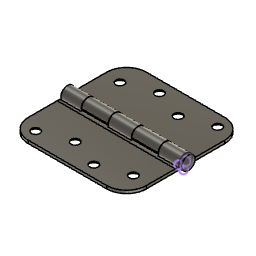
Example - Hinge v2 (Autodesk Fusion 360 design; units mm, degrees)
Autodesk Fusion 360 part; units mm, degrees
sketch "Sketch1" plane through (0, 0, 0) normal (1, 0, 0) x (0, 1, 0)
  line L0 (-56.0607, 28.9615) -> (-14.2484, 28.9615)
  line L1 (-9.4019, 28.157) -> (-6.4108, 27.1358)
  arc A0 (-6.4108, 27.1358) -> (-8.6089, 30.3207) centre (-5.3607, 30.2115) ccw
  circle A1 centre (-5.3607, 30.2115) radius 2.75
  line L2 (-56.0607, 26.4615) -> (-14.2484, 26.4615)
  line L3 (-10.2097, 25.791) -> (-7.2185, 24.7698)
  arc A2 (-7.2185, 24.7698) -> (-11.1075, 30.4047) centre (-5.3607, 30.2115) ccw
  line L4 (-56.0607, 28.9615) -> (-56.0607, 26.4615)
  line L5 (-11.1075, 30.4047) -> (-11.1411, 29.4053)
  line L6 (-11.1411, 29.4053) -> (-8.6425, 29.3212)
  line L7 (-8.6425, 29.3212) -> (-8.6089, 30.3207)
  arc A3 (-9.4019, 28.157) -> (-14.2484, 28.9615) centre (-14.2484, 13.9615) ccw
  arc A4 (-10.2097, 25.791) -> (-14.2484, 26.4615) centre (-14.2484, 13.9615) ccw
  line L8 (14.6393, 52.3652) -> (14.6393, 9.6795) construction
  arc A5 (40.386, 30.4047) -> (36.497, 24.7698) centre (34.6393, 30.2115) ccw
  circle A6 centre (34.6393, 30.2115) radius 2.75
  line L9 (85.3393, 28.9615) -> (43.5269, 28.9615)
  line L10 (85.3393, 28.9615) -> (85.3393, 26.4615)
  arc A7 (43.5269, 28.9615) -> (38.6804, 28.157) centre (43.5269, 13.9615) ccw
  line L11 (40.386, 30.4047) -> (40.4196, 29.4053)
  arc A8 (37.8874, 30.3207) -> (35.6893, 27.1358) centre (34.6393, 30.2115) ccw
  line L12 (38.6804, 28.157) -> (35.6893, 27.1358)
  line L13 (40.4196, 29.4053) -> (37.921, 29.3212)
  line L14 (39.4882, 25.791) -> (36.497, 24.7698)
  line L15 (85.3393, 26.4615) -> (43.5269, 26.4615)
  arc A9 (43.5269, 26.4615) -> (39.4882, 25.791) centre (43.5269, 13.9615) ccw
  line L16 (37.921, 29.3212) -> (37.8874, 30.3207)
  dimension "d1" = 5.5
  dimension "d3" = 50.7
  dimension "d4" = 2.5
  dimension "d5" = 1.25
  dimension "d6" = 0.5
  dimension "d7" = 2.5
  dimension "d9" = 1
  dimension "d10" = 15
  dimension "d12" = 20
  constraint tangent L1 A0
  constraint parallel L0 L2
  constraint parallel L1 L3
  constraint concentric A0 A2
  constraint tangent L3 A2
  constraint concentric A0 A1
  constraint horizontal L0
  constraint perpendicular L2 L4
  constraint tangent A2 L5
  constraint perpendicular L5 L6
  constraint perpendicular L6 L7
  constraint tangent A0 L7
  constraint tangent L0 A3
  constraint tangent L1 A3
  constraint tangent L2 A4
  constraint tangent L3 A4
  constraint concentric A3 A4
  constraint vertical L8
  constraint symmetric L0.start L8 L9.start
  constraint symmetric L1.end L8 A8.end
  constraint symmetric A0.end L8 A8.start
  constraint symmetric A0 L8 A8
  constraint symmetric A1 L8 A6
  constraint symmetric L2.start L8 L10.end
  constraint symmetric L3.end L8 A5.end
  constraint symmetric A2.end L8 A5.start
  constraint symmetric A2 L8 A5
  constraint symmetric L5.end L8 L11.end
  constraint symmetric L6.end L8 L13.end
  constraint symmetric L0.end L8 L9.end
  constraint symmetric L1.start L8 A7.end
  constraint symmetric A3 L8 A7
  constraint symmetric L2.end L8 L15.end
  constraint symmetric L3.start L8 L14.start
  constraint symmetric A4 L8 A9
  measures "d1" diameter of A1
  measures "d3" distance of A0.centre L4
  measures "d4" distance of L0 L2
  measures "d5" distance of L0 A0.centre
  measures "d6" distance of A0 A1
  measures "d7" distance of L1 L3
  measures "d9" distance of A2.end L6
  measures "d10" radius of A3
  measures "d12" distance of A0.centre L8
extrude "Extrude1" add sketch "Sketch1" along normal blind 101.4 contours L0 L1 A0 L2 L3 A2 L4 L5 L6 L7 A3 A4 makes body 1 in component "Hinge side 1"
sketch "Sketch1 (2)" plane through (0, 0, 28.9615) normal (0, 0, 1) x (-1, 0, 0) in component "Hinge side 1"
  line L0 (0, 14.2484) -> (0, 56.0607)
  line L1 (0, 56.0607) -> (-101.4, 56.0607)
  line L2 (-101.4, 56.0607) -> (-101.4, 14.2484)
  line L3 (-101.4, 14.2484) -> (0, 14.2484)
  line L4 (0, 14.2484) -> (18.3824, 20.4527)
  line L5 (18.3824, 20.4527) -> (18.3824, -4.9808)
  line L6 (18.3824, -4.9808) -> (-17.5, -4.9808)
  line L7 (-17.5, -4.9808) -> (-17.5, 14.2484)
  line L8 (-40.8, 14.2484) -> (-40.8, 11.0057)
  line L9 (-40.8, 11.0057) -> (-40.8, -4.9808)
  line L10 (-40.8, -4.9808) -> (-60.6, -4.9808)
  line L11 (-60.6, -4.9808) -> (-60.6, 14.2484)
  line L12 (-83.9, 14.2484) -> (-83.9, -4.9808)
  line L13 (-83.9, -4.9808) -> (-134.9138, -4.9808)
  line L14 (-134.9138, -4.9808) -> (-127.3022, 20.8989)
  line L15 (-127.3022, 20.8989) -> (-101.4, 14.2484)
  circle A0 centre (-13.3, 46.0607) radius 3.6
  circle A1 centre (-63.3, 46.0607) radius 3.6
  circle A2 centre (-38.3, 37.0607) radius 3.6
  circle A3 centre (-88.3, 37.0607) radius 3.6
  arc A4 (0, 39.0607) -> (-17, 56.0607) centre (-17, 39.0607) ccw
  arc A5 (-84.4, 56.0607) -> (-101.4, 39.0607) centre (-84.4, 39.0607) ccw
  line L16 (0, 11.1411) -> (0, 8.6425)
  line L17 (-60.6, 11.6411) -> (-61.7689, 11.6411)
  line L18 (0, 11.6411) -> (-83.9, 11.6411)
  arc A6 (0, 11.6411) -> (0, 13.0607) centre (0, 12.3509) ccw
  line L19 (0, 13.0607) -> (0, 14.2484)
  line L20 (-83.9, 11.6411) -> (-104.4263, 11.6411)
  line L21 (-104.4263, 11.6411) -> (-104.4263, 15.0254)
  dimension "d25" = 17.5
  dimension "d26" = 17.5
  dimension "d27" = 23.3
  dimension "d28" = 23.3
  dimension "d37" = 7.2
  dimension "d40" = -25
  dimension "d41" = -9
  dimension "d42" = 13.3
  dimension "d43" = 10
  dimension "d44" = 17
  dimension "d45" = 17
  dimension "d78" = 0.5
  constraint coincident L0.start L3.end
  constraint perpendicular L3 L5
  constraint perpendicular L0 L6
  constraint coincident L3 L7.end
  constraint perpendicular L3 L7
  constraint coincident L3 L8.start
  constraint perpendicular L3 L8
  constraint parallel L7 L9
  constraint perpendicular L7 L10
  constraint coincident L3 L11.end
  constraint perpendicular L3 L11
  constraint coincident L3 L12.start
  constraint perpendicular L3 L12
  constraint perpendicular L11 L13
  constraint coincident L2.end L3.start
  constraint collinear L6 L10
  constraint collinear L10 L13
  constraint tangent L0 A4
  constraint coincident L1 A4.end
  constraint coincident L0 A4.start
  constraint coincident L2 A5.end
  constraint coincident L1 A5.start
  constraint tangent L2 A5
  constraint tangent L1 A5
  constraint tangent L1 A4
  constraint coincident L11 L17.start
  constraint perpendicular L11 L17
  constraint coincident L12 L18.end
  constraint perpendicular L12 L18
  constraint tangent L18 A6
  constraint parallel L0 L19
  constraint perpendicular L12 L20
  constraint coincident L15 L21.end
  constraint perpendicular L20 L21
  measures "d25" distance of L0 L7
  measures "d26" distance of L2 L12
  measures "d27" distance of L7 L9
  measures "d28" distance of L11 L12
  measures "d37" diameter of A0
  measures "d42" distance of L0 A0.centre
  measures "d43" distance of L1 A0.centre
  measures "d44" radius of A5
  measures "d45" radius of A4
  measures "d78" distance of L16.start L18
extrude "Extrude2" cut sketch "Sketch1 (2)" along normal blind 10 and the other way blind 10 contours L4 L5 L6 L7 L18 A6 L19 | L0 L1 A4 | L1 L2 A5 | L8 L9 L10 L11 L18 | L12 L13 L14 L15 L20 L21 | A0 | A1 | A2 | A3 bodies 1 in component "Hinge side 1"
chamfer "Chamfer1" distance 2 angle 45 4 edges at (16.6564, -44.7589, 26.4615) (41.6564, -35.7589, 26.4615) (66.6564, -44.7589, 26.4615) (91.6564, -35.7589, 26.4615) on bodies 1 in component "Hinge side 1"
extrude "Extrude1'" add sketch "Sketch1" along normal blind 101.4 separate body contours A5 L9 L10 A7 L11 A8 L12 L13 L14 L15 A9 L16 makes body 2 in component "Hinge side 2"
sketch "Sketch1 (3)" plane through (0, 0, 28.9615) normal (0, 0, 1) x (-1, 0, 0) in component "Hinge side 2"
  line L0 (0, -85.3393) -> (0, -43.5269)
  line L1 (0, -43.5269) -> (-101.4, -43.5269)
  line L2 (-101.4, -43.5269) -> (-101.4, -85.3393)
  line L3 (-101.4, -85.3393) -> (0, -85.3393)
  line L4 (-17.75, -43.5269) -> (-17.75, -24.1924)
  line L5 (-17.75, -24.1924) -> (-40.55, -24.1924)
  line L6 (-40.55, -24.1924) -> (-40.55, -43.5269)
  line L7 (-60.85, -43.5269) -> (-60.85, -24.1924)
  line L8 (-60.85, -24.1924) -> (-83.65, -24.1924)
  line L9 (-83.65, -24.1924) -> (-83.65, -43.5269)
  line L10 (-17.5, -4.9808) -> (-17.5, 14.2484)
  line L11 (-40.8, 11.0057) -> (-40.8, -4.9808)
  line L12 (-60.6, -4.9808) -> (-60.6, 14.2484)
  line L13 (-83.9, 14.2484) -> (-83.9, -4.9808)
  line L14 (0, -40.4196) -> (0, -37.921)
  line L15 (-17.75, -40.9196) -> (-83.65, -40.9196)
  dimension "d29" = 0.25
  dimension "d30" = 0.25
  dimension "d31" = 0.25
  dimension "d32" = 0.25
  dimension "d80" = 0.5
  constraint coincident L1 L4.start
  constraint perpendicular L1 L4
  constraint perpendicular L4 L5
  constraint coincident L1 L6.end
  constraint perpendicular L1 L6
  constraint coincident L1 L7.start
  constraint perpendicular L1 L7
  constraint perpendicular L7 L8
  constraint coincident L1 L9.end
  constraint perpendicular L1 L9
  constraint coincident L4 L15.start
  constraint coincident L9 L15.end
  constraint perpendicular L9 L15
  measures "d29" distance of L4 L10
  measures "d30" distance of L6 L11
  measures "d31" distance of L7 L12
  measures "d32" distance of L9 L13
  measures "d80" distance of L14.start L15
extrude "Extrude2'" cut sketch "Sketch1 (3)" along normal blind 10 and the other way blind 10 contours L4 L5 L6 L15 | L7 L8 L9 L15 bodies 2 in component "Hinge side 2"
sketch "Sketch2" plane through (0, 0, 28.9615) normal (0, 0, 1) x (-1, 0, 0) in component "Hinge side 2"
  line L0 (0, -85.3393) -> (0, -43.5269)
  line L1 (0, -43.5269) -> (-101.4, -43.5269)
  line L2 (-101.4, -43.5269) -> (-101.4, -85.3393)
  line L3 (-101.4, -85.3393) -> (0, -85.3393)
  circle A0 centre (-13.3, -66.3393) radius 3.6
  circle A1 centre (-38.3, -75.3393) radius 3.6
  circle A2 centre (-63.3, -66.3393) radius 3.6
  circle A3 centre (-88.3, -75.3393) radius 3.6
  line L4 (0, -85.3393) -> (0, -43.5269)
  dimension "d46" = 7.2
  dimension "d47" = 7.2
  dimension "d48" = 7.2
  dimension "d49" = 7.2
  dimension "d50" = 13.3
  dimension "d51" = 25
  dimension "d52" = 50
  dimension "d53" = 50
  dimension "d54" = 10
  dimension "d55" = 19
  constraint horizontal A1.centre A3.centre
  constraint horizontal A0.centre A2.centre
  measures "d46" diameter of A0
  measures "d47" diameter of A1
  measures "d48" diameter of A2
  measures "d49" diameter of A3
  measures "d50" distance of A0.centre L4
  measures "d51" horizontal distance of A0.centre A1.centre
  measures "d52" distance of A0.centre A2.centre
  measures "d53" distance of A1.centre A3.centre
  measures "d54" distance of L3 A1.centre
  measures "d55" distance of L3 A0.centre
extrude "Extrude3" cut sketch "Sketch2" against normal blind 3 contours A0 | A1 | A2 | A3 bodies 2 in component "Hinge side 2"
chamfer "Chamfer1'" distance 2 angle 45 4 edges at (91.6564, 76.6411, 26.4615) (66.6564, 67.6411, 26.4615) (41.6564, 76.6411, 26.4615) (16.6564, 67.6411, 26.4615) on bodies 2 in component "Hinge side 2"
fillet "Fillet1" radius 17 2 edges at (0, 85.3393, 27.7115) (101.4, 85.3393, 27.7115) on bodies 2 in component "Hinge side 2"
extrude "Extrude1''" add sketch "Sketch1" along normal blind 101.4 separate body contours A1 makes body 3 in component "Hinge pin"
sketch "Sketch1 (4)" plane through (101.4, 0, 0) normal (1, 0, 0) x (0, 1, 0) in component "Hinge pin"
  circle A0 centre (-5.3607, 30.2115) radius 2.75
  arc A1 (-7.2185, 24.7698) -> (-11.1075, 30.4047) centre (-5.3607, 30.2115) ccw
  circle A2 centre (-5.3607, 30.2115) radius 5.75
  constraint concentric A1 A2
  constraint tangent A1 A2
extrude "Extrude2''" add sketch "Sketch1 (4)" along normal blind 2.5 contours A0 | A1 A2 bodies 3 in component "Hinge pin"
component "Hinge side 1" placed x (1, 0, 0) y (0, 1, 0) z (0, 0, 1) at (0, 0, 0)
component "Hinge side 2" placed x (1, 0, 0) y (0, 1, 0) z (0, 0, 1) at (0, -40, 0)
component "Hinge pin" placed x (1, 0, 0) y (0, 1, 0) z (0, 0, 1) at (0, 0, 0)
equation "d3 = ( 101.4 / 2 ) * 1 mm"
equation "d5 = d4 / 2"
equation "d7 = d4"
equation "d26 = d25"
equation "d27 = d28"
equation "d30 = d29"
equation "d31 = d29"
equation "d32 = d29"
equation "d45 = d44"
